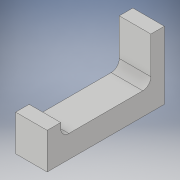
# Autodesk Inventor part: hook
Saved by Autodesk Inventor 2019 (Build 230136000, 136)
## iProperties
Created: 2018-09-20
Part Number: hook
Material: Generic
Document SubType Name: Modeling
Designer: User
Density: 1 g/cm^3
Appearance: Default
Author: User
Autodesk Inventor part; units mm, degrees
ref_plane "YZ Plane" through (0, 0, 0) normal (1, 0, 0) x (0, 1, 0)
ref_plane "XZ Plane" through (0, 0, 0) normal (0, 1, 0) x (-1, 0, 0)
ref_plane "XY Plane" through (0, 0, 0) normal (0, 0, 1) x (1, 0, 0)
sketch "Sketch1" plane through (0, 0, 0) normal (1, 0, 0) x (0, 1, 0)
  line L0 (0, 0) -> (0, -33.02)
  line L1 (0, -33.02) -> (19.05, -33.02)
  line L2 (19.05, -33.02) -> (19.05, -29.21)
  line L3 (19.05, -29.21) -> (6.35, -29.21)
  line L4 (0, 0) -> (10.16, 0)
  line L5 (10.16, 0) -> (10.16, -3.81)
  line L6 (10.16, -3.81) -> (6.35, -3.81)
  line L7 (0, 0) -> (6.35, 0)
  line L8 (6.35, -3.81) -> (6.35, -29.21)
  dimension "d0" = 33.02
  dimension "d1" = 19.05
  dimension "d2" = 3.81
  dimension "d3" = 3.81
  dimension "d4" = 10.16
  dimension "d5" = 6.35
  dimension "d6" = 6.35
  constraints: 18 end point, 5 perpendicular, 1 horizontal, 1 point on line, 1 vertical
  measures "d0" distance of L0.start L0.end
  measures "d1" distance of L0.end L1.end
  measures "d2" distance of L1.end L2.end
  measures "d3" distance of L4.end L5.end
  measures "d4" distance between parallel lines of L0 L5
  measures "d5" distance of L0.start L7.end
  measures "d6" distance between parallel lines of L0 L8
extrude "Extrusion1" add sketch "Sketch1" along normal blind 8.89
fillet "Fillet1" radius 2.286 2 edges at (4.445, 6.35, -29.21) (4.445, 6.35, -3.81)
equation "\"d3\" = d2"
body "Solid1"
